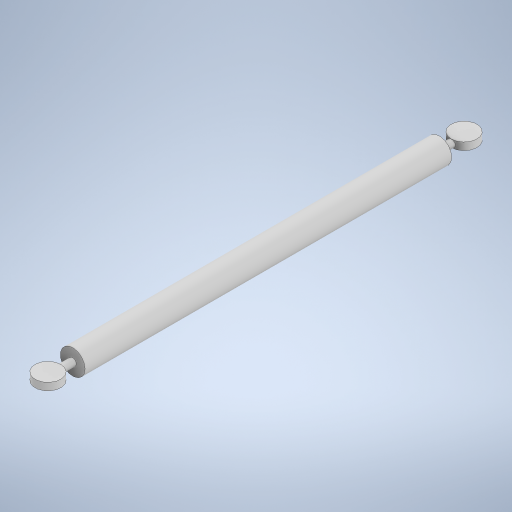
# Autodesk Inventor part: transmission_box_mount_shaft
Saved by Autodesk Inventor 2023 (Build 270158000, 158)
## iProperties
Created: 2023-09-15
Part Number: transmission_box_mount_shaft
Material: Generic
Document SubType Name: Modeling
Designer: Peter
Density: 1 g/cm^3
Appearance: Default
Author: Peter
Autodesk Inventor part; units mm, degrees
ref_plane "YZ Plane" through (0, 0, 0) normal (1, 0, 0) x (0, 1, 0)
ref_plane "XZ Plane" through (0, 0, 0) normal (0, 1, 0) x (-1, 0, 0)
sketch "Sketch1" plane through (0, 0, 0) normal (0, 0, 1) x (1, 0, 0)
  circle A0 centre (0, 0) radius 31.75
  dimension "d0" = 63.5
  constraints: 1 centre point, 1 coincident
  measures "d0" diameter of A0
extrude "Extrusion1" add sketch "Sketch1" along normal blind 939.8
sketch "Sketch2" plane through (0, 0, 0) normal (0, 0, -1) x (-1, 0, 0)
  circle A0 centre (0, 0) radius 9.525
  dimension "d3" = 19.05
  constraints: 1 centre point, 1 coincident
  measures "d3" diameter of A0
extrude "Extrusion2" add sketch "Sketch2" along normal blind 50.8
sketch "Sketch3" plane through (0, 0, 0) normal (0, 1, 0) x (-1, 0, 0)
  circle A0 centre (0, -63.5) radius 33.02
  line L0 (31.75, 0) -> (-31.75, 0) construction
  point P0 (0, 0)
  dimension "d6" = 66.04
  dimension "d7" = 63.5
  constraints: 1 centre point
  measures "d6" diameter of A0
  measures "d7" distance from line of A0.centre L0
extrude "Extrusion3" add sketch "Sketch3" along normal mid plane 19.05
ref_plane "Work Plane1" through (0, 0, 469.9) normal (0, 0, 1) x (1, 0, 0)
mirror "Mirror1" about plane through (0, 0, 469.9) normal (0, 0, 1) of "Extrusion2", "Extrusion3"
body "Solid1"
